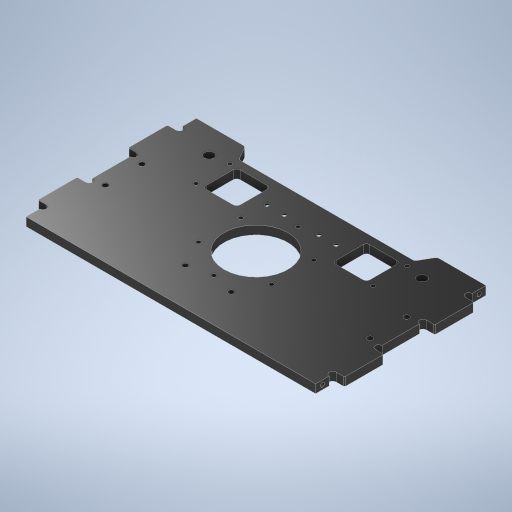
# Autodesk Inventor part: TorsoUpperFrame
Saved by Autodesk Inventor 2024.2 (Build 282272000, 272)
## iProperties
Created: 2024-01-05
Part Number: TorsoUpperFrame
Material: Aluminum 7075
Document SubType Name: Modeling
Designer: Masato Kubotera
Density: 2.81 g/cm^3
Appearance: Glossy - Black
Vendor: meviy
Mass: 108.003 g
Surface Area: 393.241 cm^2
Volume: 38.4352 cm^3
Author: Masato Kubotera
Autodesk Inventor part; units mm, degrees
ref_plane "YZ Plane" through (0, 0, 0) normal (1, 0, 0) x (0, 1, 0)
ref_plane "XZ Plane" through (0, 0, 0) normal (0, 1, 0) x (-1, 0, 0)
ref_plane "XY Plane" through (0, 0, 0) normal (0, 0, 1) x (1, 0, 0)
sketch "Sketch1" plane through (0, 0, 0) normal (0, 0, 1) x (1, 0, 0)
  line L0 (-50, -90) -> (50, -90)
  line L1 (50, -90) -> (50, 90)
  line L2 (50, 90) -> (-50, 90)
  line L3 (-50, 90) -> (-50, -90)
  line L4 (-50, -90) -> (50, 90) construction
  line L5 (50, -90) -> (-50, 90) construction
  line L6 (-50, 0) -> (50, 0)
  line L7 (0, -90) -> (0, 90) construction
  circle A0 centre (0, 0) radius 18.75
  line L8 (-12, -16) -> (31, -16) construction
  line L9 (31, -16) -> (31, 16) construction
  line L10 (31, 16) -> (-12, 16) construction
  line L11 (-12, 16) -> (-12, -16) construction
  line L12 (-12, -16) -> (31, 16) construction
  line L13 (31, -16) -> (-12, 16) construction
  line L14 (1, -13.5) -> (28, -13.5) construction
  line L15 (28, -13.5) -> (28, 13.5) construction
  line L16 (28, 13.5) -> (1, 13.5) construction
  line L17 (1, 13.5) -> (1, -13.5) construction
  line L18 (1, -13.5) -> (28, 13.5) construction
  line L19 (28, -13.5) -> (1, 13.5) construction
  line L20 (9.61, -16.1) -> (31.1, -16.1)
  line L21 (31.1, -16.1) -> (31.1, 16.1)
  line L22 (31.1, 16.1) -> (9.61, 16.1)
  line L23 (50, 85) -> (38, 85)
  line L24 (38, 85) -> (38, 90)
  line L25 (-15, 90) -> (-15, 85)
  line L26 (-15, 85) -> (15, 85)
  line L27 (15, 85) -> (15, 90)
  arc A1 (38, 85) -> (42, 85) centre (40, 85) ccw
  arc A2 (11, 85) -> (15, 85) centre (13, 85) ccw
  line L28 (-50, 85) -> (-38, 85)
  line L29 (-38, 85) -> (-38, 90)
  arc A3 (-42, 85) -> (-38, 85) centre (-40, 85) ccw
  arc A4 (-15, 85) -> (-11, 85) centre (-13, 85) ccw
  line L30 (46, 85) -> (46, 79) construction
  line L31 (-46, 85) -> (-46, 79) construction
  circle A5 centre (0, 0) radius 29 construction
  line L32 (-41.5, 0) -> (-41.5, 51.5)
  line L33 (-41.5, 51.5) -> (-50, 56.4075)
  circle A6 centre (-35, 62.5) radius 7.5 construction
  circle A7 centre (-35, 62.5) radius 5 construction
  line L34 (-70, -90.6743) -> (-70, 90) construction
  line L35 (70, -90.6743) -> (70, 90) construction
  line L36 (-50, 62.5) -> (-30, 62.5) construction
  circle A8 centre (-35, -62.5) radius 7.5 construction
  circle A9 centre (-35, -62.5) radius 5 construction
  line L37 (50, -85) -> (38, -85)
  line L38 (38, -85) -> (38, -90)
  line L39 (-15, -90) -> (-15, -85)
  line L40 (-15, -85) -> (15, -85)
  line L41 (15, -85) -> (15, -90)
  arc A10 (42, -85) -> (38, -85) centre (40, -85) ccw
  arc A11 (15, -85) -> (11, -85) centre (13, -85) ccw
  arc A12 (-11, -85) -> (-15, -85) centre (-13, -85) ccw
  line L42 (-38, -85) -> (-38, -90)
  arc A13 (-38, -85) -> (-42, -85) centre (-40, -85) ccw
  line L43 (-50, -85) -> (-38, -85)
  line L44 (-41.5, 0) -> (-41.5, -51.5)
  line L45 (-41.5, -51.5) -> (-50, -56.4075)
  line L46 (-35.6, 29.25) -> (-17.9, 29.25) construction
  line L47 (-17.4, 28.75) -> (-36.1, 28.75) construction
  line L48 (-36.6858, 30.1642) -> (-36.6858, 46.0358)
  line L49 (-35.6, 46.95) -> (-35.6, 29.25) construction
  line L50 (-35.6, 46.95) -> (-17.9, 29.25) construction
  line L51 (-17.9, 46.95) -> (-35.6, 29.25) construction
  line L52 (-36.1, 47.45) -> (-17.4, 47.45) construction
  line L53 (-36.1, 47.45) -> (-17.4, 28.75) construction
  line L54 (-17.4, 47.45) -> (-36.1, 28.75) construction
  line L55 (-36.6858, 48.0358) -> (-16.8142, 28.1642) construction
  line L56 (-16.8142, 48.0358) -> (-36.6858, 28.1642) construction
  arc A14 (-34.6858, 48.0358) -> (-36.6858, 46.0358) centre (-34.6858, 46.0358) ccw
  line L57 (-16.8142, 46.0358) -> (-16.8142, 30.1642)
  line L58 (-17.9, 29.25) -> (-17.9, 46.95) construction
  line L59 (-17.4, 47.45) -> (-17.4, 28.75) construction
  line L60 (-18.8142, 28.1642) -> (-34.6858, 28.1642)
  arc A15 (-36.6858, 30.1642) -> (-34.6858, 28.1642) centre (-34.6858, 30.1642) ccw
  arc A16 (-18.8142, 28.1642) -> (-16.8142, 30.1642) centre (-18.8142, 30.1642) ccw
  line L61 (-34.6858, 48.0358) -> (-18.8142, 48.0358)
  arc A17 (-16.8142, 46.0358) -> (-18.8142, 48.0358) centre (-18.8142, 46.0358) ccw
  line L62 (-17.9, 46.95) -> (-35.6, 46.95) construction
  line L63 (-36.1, 28.75) -> (-36.1, 47.45) construction
  line L64 (-36.6858, -30.1642) -> (-36.6858, -46.0358)
  line L65 (-34.6858, -48.0358) -> (-18.8142, -48.0358)
  line L66 (-35.6, -46.95) -> (-35.6, -29.25) construction
  line L67 (-17.9, -46.95) -> (-35.6, -46.95) construction
  line L68 (-36.1, -28.75) -> (-36.1, -47.45) construction
  line L69 (-36.1, -47.45) -> (-17.4, -47.45) construction
  line L70 (-35.6, -29.25) -> (-17.9, -29.25) construction
  line L71 (-35.6, -46.95) -> (-17.9, -29.25) construction
  line L72 (-17.9, -46.95) -> (-35.6, -29.25) construction
  line L73 (-18.8142, -28.1642) -> (-34.6858, -28.1642)
  line L74 (-16.8142, -48.0358) -> (-36.6858, -28.1642) construction
  line L75 (-36.6858, -48.0358) -> (-16.8142, -28.1642) construction
  line L76 (-17.4, -28.75) -> (-36.1, -28.75) construction
  line L77 (-36.1, -47.45) -> (-17.4, -28.75) construction
  line L78 (-17.4, -47.45) -> (-36.1, -28.75) construction
  line L79 (-17.9, -29.25) -> (-17.9, -46.95) construction
  line L80 (-17.4, -47.45) -> (-17.4, -28.75) construction
  arc A18 (-16.8142, -30.1642) -> (-18.8142, -28.1642) centre (-18.8142, -30.1642) ccw
  line L81 (-16.8142, -46.0358) -> (-16.8142, -30.1642)
  arc A19 (-34.6858, -28.1642) -> (-36.6858, -30.1642) centre (-34.6858, -30.1642) ccw
  arc A20 (-18.8142, -48.0358) -> (-16.8142, -46.0358) centre (-18.8142, -46.0358) ccw
  arc A21 (-36.6858, -46.0358) -> (-34.6858, -48.0358) centre (-34.6858, -46.0358) ccw
  arc A22 (0, 16) -> (-12, 10.583) centre (0, 0) ccw construction
  arc A23 (-12, -10.583) -> (0, -16) centre (0, 0) ccw construction
  line L82 (-26.75, 38.1) -> (-26.75, -38.1) construction
  line L83 (-14.5, 55) -> (-27.254, 55)
  arc A24 (-28.8848, 58.1579) -> (-35.7647, 69.9609) centre (-35, 62.5) ccw
  arc A25 (-28.8848, 58.1579) -> (-27.254, 55) centre (-27.254, 57) ccw
  arc A26 (-37.717, 70.9792) -> (-35.7647, 69.9609) centre (-35.9686, 71.9505) ccw
  arc A27 (-39.3295, 80) -> (-41.0778, 77.0287) centre (-39.3295, 78) ccw
  line L84 (-41.5, 16) -> (-37.5, 16) construction
  line L85 (-41.5, -16) -> (-37.5, -16) construction
  line L86 (-37.25, -49) -> (-16.25, -49) construction
  line L87 (-14.25, -47) -> (-14.25, 47) construction
  line L88 (-16.25, 49) -> (-37.25, 49) construction
  line L89 (-39.25, 47) -> (-39.25, -47) construction
  line L90 (-39.25, -49) -> (-14.25, 49) construction
  line L91 (-14.25, -49) -> (-39.25, 49) construction
  line L92 (-16.75, 52) -> (-36.75, 52) construction
  circle A28 centre (-16.75, 52) radius 1 construction
  circle A29 centre (-16.75, 52) radius 2 construction
  line L93 (-39, -55) -> (-14.5, -55) construction
  line L94 (-12.5, -53) -> (-12.5, 53) construction
  line L95 (-14.5, 55) -> (-39, 55) construction
  line L96 (-41, 53) -> (-41, -53) construction
  line L97 (-41, -55) -> (-12.5, 55) construction
  line L98 (-12.5, -55) -> (-41, 55) construction
  arc A30 (-12.5, 53) -> (-14.5, 55) centre (-14.5, 53) ccw
  arc A31 (-39, 55) -> (-41, 53) centre (-39, 53) ccw construction
  arc A32 (-41, -53) -> (-39, -55) centre (-39, -53) ccw construction
  arc A33 (-14.5, -55) -> (-12.5, -53) centre (-14.5, -53) ccw construction
  arc A34 (-37.25, 49) -> (-39.25, 47) centre (-37.25, 47) ccw construction
  arc A35 (-14.25, 47) -> (-16.25, 49) centre (-16.25, 47) ccw construction
  arc A36 (-16.25, -49) -> (-14.25, -47) centre (-16.25, -47) ccw construction
  arc A37 (-39.25, -47) -> (-37.25, -49) centre (-37.25, -47) ccw construction
  line L99 (-17.75, 22.5) -> (-35.75, 22.5) construction
  line L100 (-35.75, 22.5) -> (-35.75, -22.5) construction
  line L101 (-35.75, -22.5) -> (-17.75, -22.5) construction
  line L102 (-17.75, -22.5) -> (-17.75, 22.5) construction
  line L103 (-17.75, 22.5) -> (-35.75, -22.5) construction
  line L104 (-35.75, 22.5) -> (-17.75, -22.5) construction
  line L105 (41.0778, 77.0287) -> (13.0754, 26.6244)
  line L106 (15.6978, 25.1674) -> (43.2517, 74.7643)
  line L107 (47, 73.7931) -> (47, 3.5)
  line L108 (29.1, 18.1) -> (17.9933, 18.1)
  arc A38 (47, 73.7931) -> (43.2517, 74.7643) centre (45, 73.7931) ccw
  arc A39 (1.5, 23.4907) -> (3.2053, 21.5125) centre (3.5, 23.4907) ccw
  arc A40 (16.0474, 20.5621) -> (17.9933, 18.1) centre (17.9933, 20.1) ccw
  line L109 (-18.3808, 25.1642) -> (-34.6858, 25.1642)
  line L110 (-36.6858, 23.1642) -> (-36.6858, 0)
  arc A41 (-16.4589, 22.6106) -> (-18.3808, 25.1642) centre (-18.3808, 23.1642) ccw
  arc A42 (-34.6858, 25.1642) -> (-36.6858, 23.1642) centre (-34.6858, 23.1642) ccw
  line L111 (-34.37, -22.5) -> (-34.37, 22.5) construction
  line L112 (-29.25, 7.66) -> (-24.25, 7.66) construction
  line L113 (-24.25, 7.66) -> (-24.25, 12.66) construction
  line L114 (-24.25, 12.66) -> (-29.25, 12.66) construction
  line L115 (-29.25, 12.66) -> (-29.25, 7.66) construction
  line L116 (-29.25, 7.66) -> (-24.25, 12.66) construction
  line L117 (-24.25, 7.66) -> (-29.25, 12.66) construction
  circle A43 centre (-26.75, 10.16) radius 1.5 construction
  line L118 (-32.99, -22.5) -> (-32.99, 22.5) construction
  line L119 (-29.25, 22.82) -> (-29.25, 17.82) construction
  line L120 (-29.25, 17.82) -> (-24.25, 17.82) construction
  line L121 (-24.25, 17.82) -> (-24.25, 22.82) construction
  circle A44 centre (-26.75, 20.32) radius 1.5 construction
  line L122 (-24.25, 22.82) -> (-29.25, 22.82) construction
  arc A45 (-23.5471, 4.0762) -> (-29, 0) centre (-24.75, 0) ccw
  arc A46 (-23.5471, 4.0762) -> (-21.0458, 5.4896) centre (-22.9811, 5.9944) ccw
  arc A47 (-16.4589, 22.6106) -> (-15.3037, 18.3543) centre (-12.375, 21.4341) ccw
  arc A48 (-15.2771, 15.4814) -> (-21.0458, 5.4896) centre (0, 0) ccw
  arc A49 (-15.2771, 15.4814) -> (-15.3037, 18.3543) centre (-16.6819, 16.905) ccw
  arc A50 (5.7687, 20.971) -> (3.2053, 21.5125) centre (0, 0) ccw
  arc A51 (5.7687, 20.971) -> (8.2434, 22.4305) centre (6.2992, 22.8994) ccw
  arc A52 (11.6624, 25.624) -> (13.0754, 26.6244) centre (11.3271, 27.5956) ccw
  arc A53 (15.6978, 25.1674) -> (15.4533, 24.3645) centre (17.4462, 24.1961) ccw
  arc A54 (-3.2053, 21.5125) -> (-1.5, 23.4907) centre (-3.5, 23.4907) ccw
  line L123 (-12.5, 27.3962) -> (-12.5, 53)
  line L124 (-17, 71.5) -> (17, 71.5) construction
  line L125 (17, 71.5) -> (17, 84) construction
  line L126 (17, 84) -> (-17, 84) construction
  line L127 (-17, 84) -> (-17, 71.5) construction
  line L128 (-17, 71.5) -> (17, 84) construction
  line L129 (17, 71.5) -> (-17, 84) construction
  line L130 (-17, 77.75) -> (17, 77.75) construction
  arc A55 (-10.75, 84) -> (-10.75, 71.5) centre (-10.75, 77.75) ccw construction
  arc A56 (10.75, 71.5) -> (10.75, 84) centre (10.75, 77.75) ccw construction
  arc A57 (11.6624, 25.624) -> (8.2434, 22.4305) centre (12.375, 21.4341) ccw
  arc A58 (-3.2053, 21.5125) -> (-5.7687, 20.971) centre (0, 0) ccw
  arc A59 (-8.2434, 22.4305) -> (-5.7687, 20.971) centre (-6.2992, 22.8994) ccw
  arc A60 (-8.2434, 22.4305) -> (-11.1, 25.4884) centre (-12.375, 21.4341) ccw
  arc A61 (-12.5, 27.3962) -> (-11.1, 25.4884) centre (-10.5, 27.3962) ccw
  line L131 (17, 78) -> (17, 77.75)
  arc A62 (10.75, 71.5) -> (17, 77.75) centre (10.75, 77.75) ccw
  line L132 (10.75, 71.5) -> (3.5, 71.5)
  line L133 (-17, 78) -> (-17, 77.75)
  arc A63 (-17, 77.75) -> (-10.75, 71.5) centre (-10.75, 77.75) ccw
  line L134 (-10.75, 71.5) -> (-3.5, 71.5)
  line L135 (-39.3295, 80) -> (-19, 80)
  line L136 (19, 80) -> (39.3295, 80)
  line L137 (1.5, 23.4907) -> (1.5, 69.5)
  line L138 (-1.5, 69.5) -> (-1.5, 23.4907)
  arc A64 (-17, 78) -> (-19, 80) centre (-19, 78) ccw
  arc A65 (19, 80) -> (17, 78) centre (19, 78) ccw
  arc A66 (-1.5, 69.5) -> (-3.5, 71.5) centre (-3.5, 69.5) ccw
  arc A67 (3.5, 71.5) -> (1.5, 69.5) centre (3.5, 69.5) ccw
  arc A68 (41.0778, 77.0287) -> (39.3295, 80) centre (39.3295, 78) ccw
  line L139 (45, 1.5) -> (35.1, 1.5)
  line L140 (33.1, 3.5) -> (33.1, 14.1)
  arc A69 (45, 1.5) -> (47, 3.5) centre (45, 3.5) ccw
  arc A70 (33.1, 3.5) -> (35.1, 1.5) centre (35.1, 3.5) ccw
  arc A71 (33.1, 14.1) -> (29.1, 18.1) centre (29.1, 14.1) ccw
  line L141 (-41.0778, 77.0287) -> (-37.717, 70.9792)
  arc A72 (15.6978, 25.1674) -> (15.6898, 23.2395) centre (17.4462, 24.1961) ccw
  arc A73 (16.0474, 20.5621) -> (15.6898, 23.2395) centre (12.375, 21.4341) ccw
  point P0 (9.5, 0)
  point P1 (14.5, 0)
  point P2 (24.75, 0)
  point P3 (-12.375, -21.4341)
  point P4 (12.375, -21.4341)
  point P5 (-30, -62.5)
  point P6 (46, -85)
  point P7 (-46, -85)
  point P8 (-50, -56.4075)
  point P9 (-50, -85)
  point P10 (-38, -90)
  point P11 (-11, -85)
  point P12 (38, -90)
  point P13 (50, -85)
  point P14 (-11, 85)
  point P15 (-50, 85)
  point P16 (50, 69.4499)
  point P17 (50, 77.5499)
  point P18 (-46, -79)
  point P19 (-26.75, 38.1)
  point P20 (-26.75, 38.1)
  point P21 (-26.75, -38.1)
  point P22 (-26.75, 38.1)
  point P23 (18.75, 0)
  point P24 (-18.75, 0)
  point P25 (-35, 55)
  point P26 (-35, 70)
  point P27 (-26.75, 0)
  point P28 (-16.75, -52)
  point P29 (-36.75, -52)
  point P30 (43.8396, 82)
  point P31 (42.2091, 72.8876)
  point P32 (47, 72.8875)
  point P33 (47, 1.5)
  point P34 (33.1, 18.1)
  point P35 (-12.5, 51.9999)
  point P36 (0, 77.75)
  point P37 (1.5, 71.5)
  point P38 (-1.5, 71.5)
  point P39 (-17, 80)
  point P40 (40, 83)
  dimension "d24" = 58
  dimension "d26" = 10
  dimension "d0" = 100
  dimension "d1" = 180
  dimension "d2" = 37.5
  dimension "d3" = 43
  dimension "d4" = 32
  dimension "d5" = 27
  dimension "d6" = 27
  dimension "d7" = 9.5
  dimension "d8" = 8.5
  dimension "d9" = 0.1
  dimension "d10" = 0.1
  dimension "d15" = 360
  dimension "d17" = 49.5
  dimension "d18" = 5
  dimension "d19" = 30
  dimension "d20" = 12
  dimension "d21" = 2
  dimension "d22" = 6
  dimension "d23" = 8
  dimension "d25" = 15
  dimension "d27" = 140
  dimension "d29" = 125
  dimension "d30" = 60
  dimension "d31" = 103
  dimension "d65" = 40
  dimension "d77" = 2
  dimension "d78" = 17.7
  dimension "d79" = 17.7
  dimension "d80" = 0.5
  dimension "d81" = 76.2
  dimension "d100" = 4
  dimension "d101" = 32
  dimension "d128" = 8.5
  dimension "d130" = 29.5
  dimension "d131" = 25
  dimension "d132" = 98
  dimension "d133" = 2
  dimension "d134" = 4
  dimension "d135" = 20
  dimension "d138" = 0.5
  dimension "d139" = 6
  dimension "d140" = 2
  dimension "d141" = 2
  dimension "d149" = 18
  dimension "d150" = 45
  dimension "d151" = 2
  dimension "d153" = 3
  dimension "d157" = 3
  dimension "d160" = 2
  dimension "d161" = 3
  dimension "d173" = 15.24
  dimension "d176" = 5
  dimension "d178" = 3
  dimension "d181" = 20.32
  dimension "d184" = 10.16
  dimension "d191" = 3
  dimension "d195" = 34
  dimension "d196" = 12.5
  dimension "d197" = 1
  dimension "d205" = 5
  dimension "d206" = 3
  dimension "d212" = 2
  dimension "d213" = 3
  dimension "d215" = 4
  constraints: 284 end point, 134 point on circle, 94 point on line, 88 symmetric about line, 71 centre point, 70 tangent, 39 midpoint, 31 equal radius, 22 parallel, 21 coincident, 21 horizontal, 15 vertical, 14 perpendicular, 5 collinear, 3 horizontal alignment, 1 concentric, 49 other
  measures "d0" distance of L2.end L1.end
  measures "d1" distance of L1.end L0.end
  measures "d2" diameter of A0
  measures "d3" distance of L10.end L9.end
  measures "d4" distance of L9.end L8.end
  measures "d5" distance of L16.end L15.end
  measures "d6" distance of L15.end L14.end
  measures "d7" distance from line of point (9.5, 0) L7
  measures "d8" distance from line of point (9.5, 0) L17
  measures "d9" distance between parallel lines of L22 L10
  measures "d10" distance between parallel lines of L21 L9
  measures "d17" distance of point (24.75, 0) point (-24.75, 0)
  measures "d18" distance between parallel lines of L2 L23
  measures "d19" distance between parallel lines of L27 L25
  measures "d20" distance from line of L1.end L24
  measures "d21" radius of A1
  measures "d22" distance of L30.start L30.end
  measures "d23" distance between parallel lines of L30 L24
  measures "d25" diameter of A6
  measures "d27" distance between parallel lines of L35 L34
  measures "d29" distance of point (-35, 62.5) point (-35, -62.5)
  measures "d30" angle of L32 L33
  measures "d31" distance of L44.end L32.end
  measures "d65" distance from line of L36.end L34
  measures "d77" radius of A15
  measures "d78" distance of L46.end L49.end
  measures "d79" distance of L49.end L49.start
  measures "d80" distance between parallel lines of L49 L63
  measures "d81" distance of L82.end point (-26.75, 38.1)
  measures "d100" distance of L84.start L84.end
  measures "d101" distance between parallel lines of L85 L84
  measures "d128" distance between parallel lines of L32 L3
  measures "d130" distance between parallel lines of L11 L32
  measures "d131" distance of L91.end L90.end
  measures "d132" distance of L90.end L91.start
  measures "d133" diameter of A28
  measures "d134" diameter of A29
  measures "d135" distance of L92.start L92.end
  measures "d138" distance between parallel lines of L94 L11
  measures "d139" distance between parallel lines of L95 L88
  measures "d140" radius of A30
  measures "d141" radius of A34
  measures "d149" distance of L101.end L100.end
  measures "d150" distance of L100.end L99.end
  measures "d151" distance between parallel lines of L108 L22
  measures "d153" distance between parallel lines of L106 L105
  measures "d157" distance between parallel lines of L1 L107
  measures "d160" radius of A41
  measures "d161" distance between parallel lines of L60 L109
  measures "d173" diameter of L111 L82
  measures "d176" distance of L114.end L113.end
  measures "d178" diameter of A43
  measures "d181" diameter of A43.centre L6
  measures "d184" distance of L114.end L119.start
  measures "d191" radial gap between concentric circles of A0 A48
  measures "d195" distance of L126.end L125.end
  measures "d196" distance of L125.end L124.end
  measures "d197" distance between parallel lines of L126 L26
  measures "d205" distance of L112.end L113.end
  measures "d206" distance between parallel lines of L138 L137
  measures "d212" distance between parallel lines of L21 L140
  measures "d213" diameter of L139 L6
  measures "d215" radius of A71
extrude "Extrusion1" add sketch "Sketch1" along normal blind 5 contours L3 L28 A3 L29 L2 L25 A4 L26 A2 L27 L24 A1 L23 L1 L6 L21 L22 A0 A45 A46 A48 A49 A47 A41 L109 A42 L110 L32 L33 | L110 A42 L109 A41 A47 A49 A48 A46 A45 L6 | L6 A0 L22 L21 | L83 A25 A24 A26 L141 A27 L135 A64 L133 A63 L134 A66 L138 A54 A58 A59 A60 A61 L123 A30 | L105 A52 A57 A51 A50 A39 L137 A67 L132 A62 L131 A65 L136 A68 | L106 A38 L107 A69 L139 A70 L140 A71 L108 A40 A73 A72 A53
extrude "Extrusion2" cut sketch "Sketch1" along normal blind 2 contours L21 L20 A0 L6 | L6 A0 L22 L21
extrude "Extrusion3" cut sketch "Sketch1" along normal blind 4 contours L110 A42 L109 A41 A47 A49 A48 A46 A45 L6 | L83 A25 A24 A26 L141 A27 L135 A64 L133 A63 L134 A66 L138 A54 A58 A59 A60 A61 L123 A30 | L105 A52 A57 A51 A50 A39 L137 A67 L132 A62 L131 A65 L136 A68 | L106 A38 L107 A69 L139 A70 L140 A71 L108 A40 A73 A72 A53
hole "M3" at (12.375, -21.4341, 0) at (24.75, 0, 0) at (12.375, 21.4341, 0) at (-12.375, 21.4341, 0) at (-12.375, -21.4341, 0) at (-24.75, 0, 0) at (-35, -62.5, 0) at (-26.75, 10.16, 0) at (-26.75, 20.32, 0) direction (0, 0, 1) diameter 2.459 end through all thread size "M3x0.5" class "6H" standard "ANSI Metric M Profile"
hole "M4" at (-10.75, 77.75, 0) at (10.75, 77.75, 0) direction (0, 0, 1) diameter 3.242 end through all thread size "M4x0.7" class "6H" standard "ANSI Metric M Profile"
hole "Phi3.1" at (28, -13.5, 0) at (28, 13.5, 0) direction (0, 0, 1) diameter 3.1 end through all
hole "Phi5.5" at (-35, 62.5, 0) at (-35, -62.5, 0) direction (0, 0, 1) diameter 5.5 end through all
sketch "Sketch2" plane through (-11, 85, 0) normal (0, 1, 0) x (1, 0, 0)
  line L0 (44, 0) -> (53, 0) projected
  line L1 (57, 0) -> (57, -5) construction
  line L2 (61, -5) -> (53, -5) projected
  line L3 (61, 0) -> (53, 0) projected
  line L4 (-31, -5) -> (-39, -5) projected
  line L5 (-35, -5) -> (-35, 0) construction
  point P0 (11, 0)
  point P1 (57, -2.5)
  point P2 (-35, -2.5)
  point P3 (-35, 0)
  point P4 (57, 0)
  point P5 (57, -2.5)
  point P6 (-35, -2.5)
  constraints: 5 midpoint, 4 end point, 3 coincident, 2 vertical
hole "Side-M3" at (46, 85, 2.5) at (-46, 85, 2.5) direction (0, -1, 0) diameter 2.459 depth 6 thread size "M3x0.5" class "6H" standard "ANSI Metric M Profile"
hole "Phi2.5" at (-16.75, 52, 0) at (-36.75, 52, 0) at (-16.75, -52, 0) at (-36.75, -52, 0) direction (0, 0, 1) diameter 2.5 end through all
fillet "R2" radius 2 3 edges at (31.1, 16.1, 1) (-41.5, 51.5, 2.5) (-50, 56.4075, 2.5)
chamfer "C0.5" distance 0.5 angle 45 4 edges at (38, 90, 2.5) (15, 90, 2.5) (-15, 90, 2.5) (-38, 90, 2.5)
mirror "Mirror1" about plane through (0, 0, 0) normal (0, 1, 0)
sketch "Sketch3" plane through (-41.5, 50.3453, 0) normal (-1, 0, 0) x (0, 0, 1)
  line L0 (5, 0) -> (5, -100.6906) projected
  line L1 (5, -34.3453) -> (0, -34.3453)
  line L2 (5, -66.3453) -> (0, -66.3453)
  point P0 (0, -50.3453)
  point P1 (2.5, -34.3453)
  point P2 (0, -66.3453)
  point P3 (2.5, -66.3453)
  constraints: 4 end point, 2 coincident, 2 horizontal, 2 midpoint, 2 point on line
hole "Side-M2" [suppressed]
equation "\"d10\" = d9"
body "Solid1"
